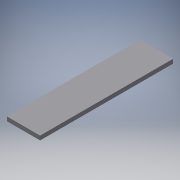
# Autodesk Inventor part: Drive Motor Plate
Saved by Autodesk Inventor 2017 (Build 210142000, 142)
## iProperties
Created: 2016-12-03
Part Number: Drive Motor Plate
Material: Generic
Document SubType Name: Modeling
Designer: Aditya
Density: 1 g/cm^3
Appearance: Default
Author: Aditya
Autodesk Inventor part; units mm, degrees
ref_plane "YZ Plane" through (0, 0, 0) normal (1, 0, 0) x (0, 1, 0)
ref_plane "XZ Plane" through (0, 0, 0) normal (0, 1, 0) x (-1, 0, 0)
ref_plane "XY Plane" through (0, 0, 0) normal (0, 0, 1) x (1, 0, 0)
sketch "Sketch1" plane through (0, 0, 0) normal (0, 1, 0) x (-1, 0, 0)
  line L0 (0, 0) -> (0, -101.6)
  line L1 (0, -101.6) -> (25.4, -101.6)
  line L2 (25.4, -101.6) -> (25.4, 0)
  line L3 (25.4, 0) -> (0, 0)
  dimension "d0" = 101.6
  dimension "d1" = 25.4
  constraints: 8 end point, 2 perpendicular, 2 vertical
  measures "d0" distance of L0.start L0.end
  measures "d1" distance of L0.end L1.end
extrude "Extrusion1" add sketch "Sketch1" along normal blind 3.175
body "Solid1"
